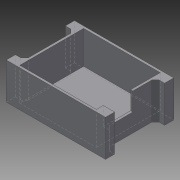
# Autodesk Inventor part: main body
Saved by Autodesk Inventor 2015 (Build 190159000, 159)
## iProperties
Created: 2019-05-11
Part Number: main body
Material: Generic
Document SubType Name: Modeling
Designer: Toby
Density: 1 g/cm^3
Appearance: Default
Author: Toby
Autodesk Inventor part; units mm, degrees
ref_plane "YZ Plane" through (0, 0, 0) normal (1, 0, 0) x (0, 1, 0)
ref_plane "XZ Plane" through (0, 0, 0) normal (0, 1, 0) x (-1, 0, 0)
ref_plane "XY Plane" through (0, 0, 0) normal (0, 0, 1) x (1, 0, 0)
sketch "Sketch1" plane through (0, 0, 0) normal (0, 0, 1) x (1, 0, 0)
  line L0 (-36.3054, 10.7035) -> (5.6946, 10.7035)
  line L1 (5.6946, 10.7035) -> (5.6946, -24.2965)
  line L2 (5.6946, -24.2965) -> (-36.3054, -24.2965)
  line L3 (-36.3054, -24.2965) -> (-36.3054, 10.7035)
  line L4 (-37.5054, 11.9035) -> (6.8946, 11.9035)
  line L5 (6.8946, 11.9035) -> (6.8946, -25.4965)
  line L6 (6.8946, -25.4965) -> (-37.5054, -25.4965)
  line L7 (-37.5054, -25.4965) -> (-37.5054, 11.9035)
  point P0 (0, 0)
  dimension "d0" = 42
  dimension "d1" = 35
  dimension "d2" = 1.2
  dimension "d3" = 1.2
  dimension "d4" = 1.2
  dimension "d5" = 1.2
  constraints: 16 end point, 4 parallel, 2 horizontal, 2 perpendicular
  measures "d0" distance of L0.start L0.end
  measures "d1" distance of L2.end L0.start
  measures "d2" distance between parallel lines of L0 L4
  measures "d3" distance between parallel lines of L6 L2
  measures "d4" distance between parallel lines of L7 L3
  measures "d5" distance between parallel lines of L5 L1
extrude "Extrusion1" add sketch "Sketch1" along normal blind 18
sketch "Sketch2" plane through (0, 0, 0) normal (0, 0, -1) x (-1, 0, 0)
  line L0 (-11.8946, 11.9035) -> (42.5054, 11.9035)
  line L1 (42.5054, 11.9035) -> (42.5054, -25.4965)
  line L2 (42.5054, -25.4965) -> (-11.8946, -25.4965)
  line L3 (-11.8946, -25.4965) -> (-11.8946, 11.9035)
  line L4 (-6.8946, -25.4965) -> (-6.8946, 11.9035) projected
  line L5 (37.5054, -25.4965) -> (37.5054, 11.9035) projected
  line L6 (37.5054, 11.9035) -> (-6.8946, 11.9035) projected
  line L7 (-6.8946, -25.4965) -> (37.5054, -25.4965) projected
  point P0 (0, 0)
  dimension "d8" = 5
  dimension "d9" = 5
  constraints: 8 end point, 2 collinear, 2 parallel, 1 horizontal, 1 perpendicular
  measures "d8" distance between parallel lines of L4 L3
  measures "d9" distance between parallel lines of L1 L5
extrude "Extrusion2" add sketch "Sketch2" along normal blind 2
sketch "Sketch3" plane through (0, 0, 0) normal (0, 0, 1) x (1, 0, 0)
  line L0 (-42.5054, 11.9035) -> (11.8946, 11.9035) projected
  line L1 (-42.5054, -25.4965) -> (-42.5054, 11.9035) projected
  line L2 (-37.5054, 11.9035) -> (-42.5054, 11.9035)
  line L3 (-42.5054, 11.9035) -> (-42.5054, 6.9035)
  line L4 (-42.5054, 6.9035) -> (-37.5054, 6.9035)
  line L5 (-37.5054, 6.9035) -> (-37.5054, 11.9035)
  line L6 (-37.5054, 11.9035) -> (-37.5054, -25.4965) projected
  line L7 (-42.5054, -25.4965) -> (-37.5054, -25.4965)
  line L8 (-37.5054, -25.4965) -> (-37.5054, -20.4965)
  line L9 (-37.5054, -20.4965) -> (-42.5054, -20.4965)
  line L10 (-42.5054, -20.4965) -> (-42.5054, -25.4965)
  line L11 (6.8946, 11.9035) -> (6.8946, -25.4965) projected
  line L12 (11.8946, 11.9035) -> (6.8946, 11.9035)
  line L13 (6.8946, 11.9035) -> (6.8946, 6.9035)
  line L14 (6.8946, 6.9035) -> (11.8946, 6.9035)
  line L15 (11.8946, 6.9035) -> (11.8946, 11.9035)
  line L16 (11.8946, -25.4965) -> (6.8946, -25.4965)
  line L17 (6.8946, -25.4965) -> (6.8946, -20.4965)
  line L18 (6.8946, -20.4965) -> (11.8946, -20.4965)
  line L19 (11.8946, -20.4965) -> (11.8946, -25.4965)
  point P0 (0, 0)
  dimension "d12" = 5
  dimension "d13" = 5
  dimension "d14" = 5
  dimension "d15" = 5
  constraints: 32 end point, 8 parallel, 5 point on line, 4 horizontal, 4 perpendicular, 1 collinear
  measures "d12" distance of L3.end L2.end
  measures "d13" distance of L8.end L7.end
  measures "d14" distance of L13.end L12.end
  measures "d15" distance of L17.end L18.end
extrude "Extrusion3" add sketch "Sketch3" along normal blind 18 contours L0 L5 L4 L1 | L9 L6 L7 L1 | L0 L15 L14 L11 | L18 L19 L16 L11
sketch "Sketch4" plane through (0, 0, 0) normal (0, 0, 1) x (1, 0, 0)
  line L0 (-37.5054, 6.9035) -> (-42.5054, 6.9035)
  line L1 (-42.5054, 6.9035) -> (-42.5054, -20.4965)
  line L2 (-42.5054, -20.4965) -> (-37.5054, -20.4965)
  line L3 (-37.5054, -20.4965) -> (-37.5054, 6.9035)
  line L4 (6.8946, -20.4965) -> (11.8946, -20.4965)
  line L5 (11.8946, -20.4965) -> (11.8946, 6.9035)
  line L6 (11.8946, 6.9035) -> (6.8946, 6.9035)
  line L7 (6.8946, 6.9035) -> (6.8946, -20.4965)
  point P0 (0, 0)
  constraints: 16 end point, 4 parallel, 2 horizontal, 2 perpendicular
extrude "Extrusion4" cut sketch "Sketch4" against normal blind 18
chamfer "Chamfer1" distance 2 angle 45 4 edges at (-37.5054, 6.9035, 8) (-37.5054, -20.4965, 8) (6.8946, 6.9035, 8) (6.8946, -20.4965, 8)
sketch "Sketch5" plane through (0, 0, 18) normal (0, 0, 1) x (1, 0, 0)
  line L0 (5.6946, 10.7035) -> (5.6946, -24.2965) projected
  line L1 (8.8946, -20.4965) -> (5.6946, -20.4965)
  line L2 (5.6946, -20.4965) -> (5.6946, -5.4965)
  line L3 (5.6946, -5.4965) -> (8.8946, -5.4965)
  line L4 (8.8946, -5.4965) -> (8.8946, -20.4965)
  point P0 (0, 0)
  dimension "d23" = 15
  constraints: 8 end point, 2 parallel, 1 horizontal, 1 perpendicular, 1 point on line
  measures "d23" distance of L1.end L2.end
extrude "Extrusion5" cut sketch "Sketch5" against normal blind 10
body "Solid1"
